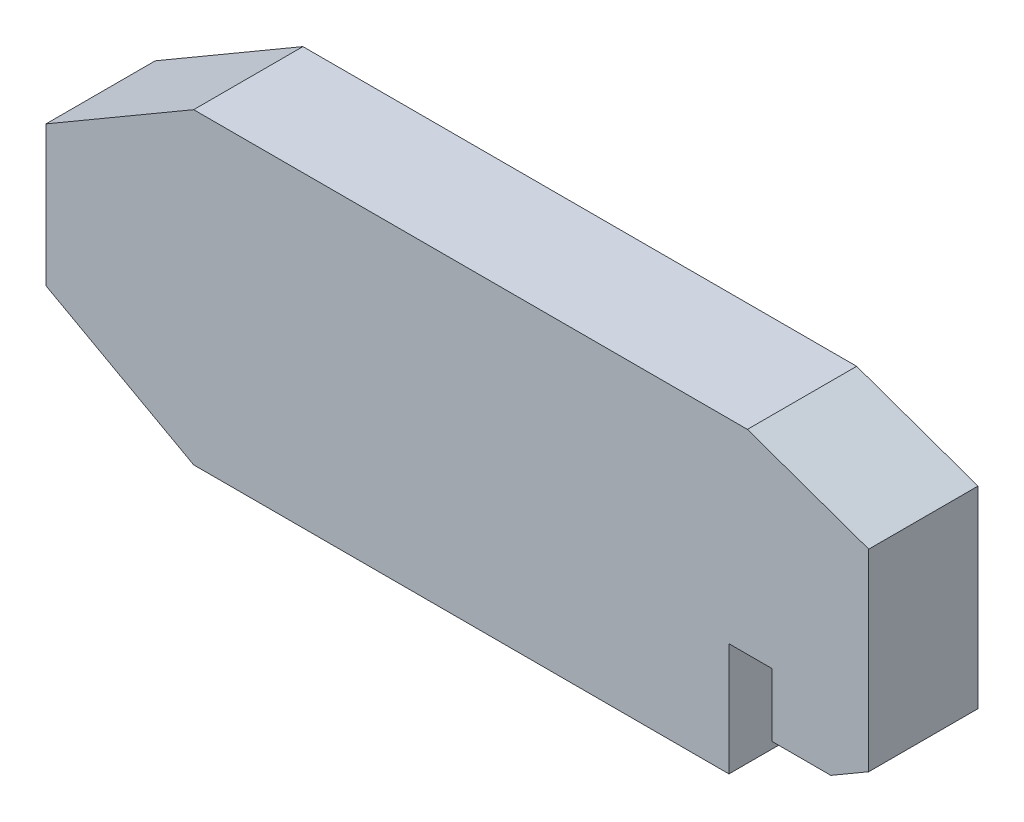
# Autodesk Inventor part: flatcamera
Saved by Autodesk Inventor 2020 (Build 240168000, 168)
## iProperties
Created: 2019-10-31
Part Number: flatcamera
Material: Generic
Document SubType Name: Modeling
Designer: Hymowitz
Density: 1 g/cm^3
Appearance: Default
Author: Hymowitz
Autodesk Inventor part; units mm, degrees
ref_plane "YZ Plane" through (0, 0, 0) normal (1, 0, 0) x (0, 1, 0)
ref_plane "XZ Plane" through (0, 0, 0) normal (0, 1, 0) x (-1, 0, 0)
ref_plane "XY Plane" through (0, 0, 0) normal (0, 0, 1) x (1, 0, 0)
sketch "Sketch1" plane through (0, 0, 0) normal (0, 0, 1) x (1, 0, 0)
  line L0 (-91.2456, 87.8277) -> (124.6544, 87.8277) construction
  line L1 (124.6544, 87.8277) -> (124.6544, -191.7916) construction
  line L2 (124.6544, -191.7916) -> (-91.2456, -191.7916) construction
  line L3 (-91.2456, -191.7916) -> (-91.2456, 87.8277) construction
  line L4 (-40.6804, 60.9272) -> (-30.3811, 66.9352)
  line L5 (-30.3811, 66.9352) -> (8.2414, 66.9352)
  line L6 (8.2414, 66.9352) -> (16.7044, 63.9312)
  line L7 (16.7044, 63.9312) -> (16.7044, 50.4848)
  line L8 (16.7044, 50.4848) -> (14.0633, 48.9442)
  line L9 (14.0633, 48.9442) -> (9.958, 48.9442)
  line L10 (9.958, 48.9442) -> (9.958, 53.3458)
  line L11 (9.958, 53.3458) -> (6.954, 53.3458)
  line L12 (6.954, 53.3458) -> (6.954, 45.4782)
  line L13 (6.954, 45.4782) -> (-30.3811, 45.4782)
  line L14 (-40.6804, 51.145) -> (-40.6804, 60.9272)
  line L15 (-30.3811, 45.4782) -> (-40.6804, 51.145)
  point P0 (0, 0)
  dimension "d4" = 215.9
  constraints: 24 end point, 5 perpendicular, 2 horizontal, 1 parallel, 1 vertical, 2 other
  measures "d4" distance of L0.start L0.end
extrude "Extrusion1" add sketch "Sketch1" along normal blind 7.62
body "Solid1"
